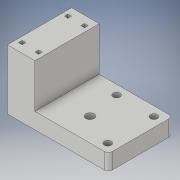
# Autodesk Inventor part: BaseMount
Saved by Autodesk Inventor 2019 (Build 230136000, 136)
## iProperties
Created: 2019-06-10
Part Number: BaseMount
Material: Generic
Document SubType Name: Modeling
Designer: aorfi
Density: 1 g/cm^3
Appearance: Default
Author: aorfi
Autodesk Inventor part; units mm, degrees
ref_plane "YZ Plane" through (0, 0, 0) normal (1, 0, 0) x (0, 1, 0)
ref_plane "XZ Plane" through (0, 0, 0) normal (0, 1, 0) x (-1, 0, 0)
ref_plane "XY Plane" through (0, 0, 0) normal (0, 0, 1) x (1, 0, 0)
sketch "Sketch1" plane through (0, 0, 0) normal (0, 1, 0) x (-1, 0, 0)
  line L0 (-27.5, 17.5) -> (27.5, 17.5)
  line L1 (27.5, 17.5) -> (27.5, -17.5)
  line L2 (27.5, -17.5) -> (-27.5, -17.5)
  line L3 (-27.5, -17.5) -> (-27.5, 17.5)
  line L4 (-27.5, 17.5) -> (27.5, -17.5) construction
  line L5 (27.5, 17.5) -> (-27.5, -17.5) construction
  point P0 (0, 0)
  dimension "d0" = 35
  dimension "d1" = 55
  constraints: 12 end point, 2 midpoint, 2 parallel, 1 horizontal, 1 perpendicular
  measures "d0" distance of L0.end L1.end
  measures "d1" distance of L1.end L2.end
extrude "Extrusion1" add sketch "Sketch1" along normal mid plane 8.763
sketch "Sketch2" plane through (0, 4.3815, 0) normal (0, 1, 0) x (1, 0, 0)
  line L0 (-27.5, -17.5) -> (27.5, -17.5) projected
  line L1 (27.5, -17.5) -> (27.5, 17.5) projected
  point P0 (4.8, -4.8)
  dimension "d11" = 12.7
  dimension "d12" = 22.7
  measures "d11" distance from line of L0 point (4.8, -4.8)
  measures "d12" distance from line of L1 point (4.8, -4.8)
hole "Hole1" at (4.8, 4.3815, 4.8) direction (0, -1, 0) diameter 4.496 end through all clearance for "Flat Head Machine Screw (82)" size "#8" standard "Ansi Unified Screw Threads"
sketch "Sketch3" plane through (0, 4.3815, 0) normal (0, 1, 0) x (1, 0, 0)
  line L0 (27.5, 17.5) -> (-27.5, 17.5) projected
  line L1 (-27.5, 17.5) -> (-12.5, 17.5)
  line L2 (-12.5, 17.5) -> (-12.5, -17.5)
  line L3 (-12.5, -17.5) -> (-27.5, -17.5)
  line L4 (-27.5, -17.5) -> (-27.5, 17.5)
  line L5 (-27.5, -17.5) -> (27.5, -17.5) projected
  point P0 (0, 0)
  dimension "d13" = 15
  constraints: 8 end point, 2 parallel, 1 collinear, 1 horizontal, 1 perpendicular
  measures "d13" distance of L2.end L3.end
extrude "Extrusion2" add sketch "Sketch3" along normal blind 23.897
sketch "Sketch9" plane through (0, -4.3815, 0) normal (0, -1, 0) x (1, 0, 0)
  circle A0 centre (4.8, 4.8) radius 2.248 projected
  circle A1 centre (4.8, 4.8) radius 4
  point P0 (0, 0)
  dimension "d40" = 8
  constraints: 1 centre point, 1 coincident
  measures "d40" diameter of A1
extrude "Extrusion8" cut sketch "Sketch9" against normal blind 4.318
sketch "Sketch10" plane through (0, -4.3815, 0) normal (0, -1, 0) x (1, 0, 0)
  line L0 (27.5, -17.5) -> (27.5, 17.5) projected
  line L1 (-27.5, -17.5) -> (27.5, -17.5) projected
  point P0 (0, 0)
  point P1 (22.42, -12.42)
  point P2 (22.42, 12.726)
  point P3 (2.1, -12.42)
  dimension "d43" = 5.08
  dimension "d44" = 5.08
  dimension "d45" = 20.32
  dimension "d46" = 25.146
  constraints: 1 horizontal alignment, 1 vertical alignment
  measures "d43" distance from line of L0 point (22.42, -12.42)
  measures "d44" distance from line of L1 point (22.42, -12.42)
  measures "d45" distance of point (2.1, -12.42) point (22.42, -12.42)
  measures "d46" distance of point (22.42, -12.42) point (22.42, 12.726)
hole "Hole2" at (22.42, -4.3815, -12.42) at (22.42, -4.3815, 12.726) at (2.1, -4.3815, -12.42) direction (0, 1, 0) diameter 3.797 end through all clearance for "Flat Head Machine Screw (82)" size "#6" standard "Ansi Unified Screw Threads"
fillet "Fillet1" radius 2 2 edges at (27.5, 0, 17.5) (27.5, 0, -17.5)
sketch "Sketch11" plane through (0, 28.2785, 0) normal (0, 1, 0) x (1, 0, 0)
  line L0 (-25.5, 13.5) -> (-23.5, 13.5)
  line L1 (-23.5, 13.5) -> (-23.5, 11.5)
  line L2 (-23.5, 11.5) -> (-25.5, 11.5)
  line L3 (-25.5, 11.5) -> (-25.5, 13.5)
  line L4 (-14.5, 13.5) -> (-16.5, 13.5)
  line L5 (-16.5, 13.5) -> (-16.5, 11.5)
  line L6 (-16.5, 11.5) -> (-14.5, 11.5)
  line L7 (-14.5, 11.5) -> (-14.5, 13.5)
  line L8 (-25.5, -11.5) -> (-23.5, -11.5)
  line L9 (-23.5, -11.5) -> (-23.5, -13.5)
  line L10 (-23.5, -13.5) -> (-25.5, -13.5)
  line L11 (-25.5, -13.5) -> (-25.5, -11.5)
  line L12 (-14.5, -11.5) -> (-16.5, -11.5)
  line L13 (-16.5, -11.5) -> (-16.5, -13.5)
  line L14 (-16.5, -13.5) -> (-14.5, -13.5)
  line L15 (-14.5, -13.5) -> (-14.5, -11.5)
  line L16 (-24.5, 12.5) -> (-15.5, 12.5) construction
  line L17 (-12.5, 17.5) -> (-27.5, 17.5) construction
  line L18 (-24.5, 12.5) -> (-24.5, -12.5) construction
  line L19 (-27.5, 17.5) -> (-27.5, -17.5) projected
  point P0 (0, 0)
  point P1 (-24.5, 13.5)
  point P2 (-15.5, 13.5)
  point P3 (-20, 12.5)
  point P4 (-20, 17.5)
  point P5 (-25.5, 12.5)
  point P6 (-25.5, -12.5)
  point P7 (-27.5, 0)
  point P8 (-24.5, 0)
  dimension "d57" = 2
  dimension "d58" = 2
  dimension "d59" = 2
  dimension "d60" = 2
  dimension "d61" = 5
  dimension "d62" = 3
  constraints: 36 end point, 8 midpoint, 8 parallel, 6 collinear, 5 horizontal, 4 perpendicular, 3 point on line, 3 vertical alignment, 2 horizontal alignment, 1 vertical
  measures "d57" distance of L0.start L0.end
  measures "d58" distance of L2.end L0.start
  measures "d59" distance of L4.start L4.end
  measures "d60" distance of L10.end L8.start
  measures "d61" distance between parallel lines of L17 L16
  measures "d62" distance between parallel lines of L19 L18
extrude "Extrusion9" cut sketch "Sketch11" against normal blind 3
equation "\"d44\" = d43"
equation "\"d58\" = d57"
equation "\"d59\" = d57"
equation "\"d60\" = d57"
body "Solid1"
